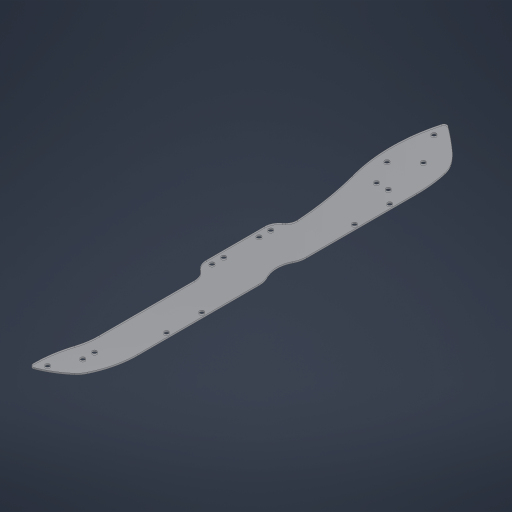
# Autodesk Inventor part: sled2
Saved by Autodesk Inventor 2024 (Build 280153000, 153)
## iProperties
Created: 2023-10-30
Part Number: sled2
Material: Polycarbonate, Smoke
Document SubType Name: Modeling
Designer: macbook
Density: 1.2 g/cm^3
Appearance: Polycarbonate - Clear(1)
Author: macbook
Autodesk Inventor part; units mm, degrees
ref_plane "YZ Plane" through (0, 0, 0) normal (1, 0, 0) x (0, 1, 0)
ref_plane "XZ Plane" through (0, 0, 0) normal (0, 1, 0) x (-1, 0, 0)
ref_plane "XY Plane" through (0, 0, 0) normal (0, 0, 1) x (1, 0, 0)
sketch "Sketch2" plane through (0, 0, 0) normal (0, 1, 0) x (-1, 0, 0)
  line L0 (25.3485, -88.9331) -> (25.3485, -76.2331)
  line L1 (25.3485, -76.2331) -> (0.0063, -76.2331)
  line L2 (0.0063, -76.2331) -> (0.0055, -63.5331)
  line L3 (0.1328, -20.6833) -> (0.1265, -35.8822)
  line L4 (38.2012, -93.5899) -> (38.2012, -99.9399)
  line L5 (12.8495, -23.9499) -> (19.1995, -23.9501)
  line L6 (19.1995, -23.9501) -> (6.4995, -23.9497)
  line L7 (25.3485, -88.9331) -> (31.6373, -88.0533)
  arc A0 (30.6963, -113.4359) -> (33.2246, -115.3327) centre (248.7957, 174.6442) ccw
  line L8 (38.2825, -88.8911) -> (38.2774, -69.8411)
  line L9 (38.2774, -69.8411) -> (44.78, -69.8393)
  arc A1 (38.3114, -113.5855) -> (38.3007, -17.4758) centre (-135.3855, -65.5498) ccw
  arc A2 (33.2246, -115.3327) -> (38.3114, -113.5855) centre (35.1695, -112.7166) ccw
  arc A3 (44.8311, -65.5299) -> (38.2642, -32.0968) centre (-43.6087, -65.5397) ccw
  line L10 (6.4995, -23.9497) -> (0.1314, -23.947)
  line L11 (0.1314, -23.947) -> (0.2658, 299.9029) construction
  line L12 (0.2658, 299.9029) -> (25.6658, 299.9029) construction
  line L13 (25.6658, 269.4446) -> (25.6658, -23.6933)
  line L14 (25.6658, -23.6933) -> (39.903, -23.6933)
  line L15 (0.2658, 299.9029) -> (-12.4342, 299.9029)
  line L16 (-12.5436, -23.9601) -> (-12.5436, -35.112)
  arc A4 (-4.3142, -80.5045) -> (7.2064, -94.0414) centre (51.9465, -44.2947) ccw
  arc A5 (-12.5436, -35.112) -> (-9.0134, -68.7415) centre (149.4014, -35.112) ccw
  arc A6 (-5.9833, -77.5413) -> (-4.3142, -80.5045) centre (19.9766, -64.8707) ccw
  arc A7 (-9.0134, -68.7415) -> (-5.9833, -77.5413) centre (28.2561, -60.8297) ccw
  arc A8 (7.2064, -94.0414) -> (30.6963, -113.4359) centre (248.7971, 174.6431) ccw
  line L17 (0.2658, 299.9029) -> (0.1867, 109.403) construction
  line L18 (0.1867, 109.403) -> (-36.5163, 109.4182)
  arc A9 (-9.714, 95.5829) -> (-9.702, 123.2303) centre (-36.5163, 109.4182) ccw
  line L19 (-12.5217, 258.1981) -> (-12.5217, 134.8616)
  line L20 (-12.5436, 83.9322) -> (-12.5436, -23.9601)
  arc A10 (-12.5217, 127.6948) -> (-12.5436, 91.1127) centre (-36.5163, 109.4182) ccw construction
  arc A11 (-12.5217, 134.8616) -> (-9.702, 123.2303) centre (12.8783, 134.8616) ccw
  arc A12 (-9.714, 95.5829) -> (-12.5436, 83.9322) centre (12.8564, 83.9322) ccw
  line L21 (25.6658, 299.9029) -> (25.6658, 331.6529)
  line L22 (25.6658, 331.6529) -> (32.0158, 331.6529)
  arc A13 (35.1908, 331.6395) -> (28.8408, 331.6529) centre (32.0158, 331.6529) ccw
  line L23 (0.2658, 299.9029) -> (0.2658, 325.3029)
  line L24 (32.0158, 331.6529) -> (30.6929, 331.6529)
  arc A14 (29.2214, 292.4497) -> (35.1908, 331.6395) centre (-92.7618, 331.0796) ccw
  line L25 (31.9383, 334.827) -> (31.4142, 334.827)
  arc A15 (31.007, 334.6634) -> (4.0007, 318.3551) centre (65.1249, 247.6497) ccw
  arc A16 (-10.3215, 302.8155) -> (-14.0041, 295.5815) centre (10.1821, 287.8234) ccw
  line L26 (-12.5217, 258.1981) -> (-12.5217, 338.0406)
  arc A17 (-2.1991, 310.3119) -> (-12.5217, 265.7661) centre (88.7553, 265.7661) ccw
  arc A18 (4.0007, 318.3551) -> (-2.1991, 310.3119) centre (20.612, 299.1399) ccw
  line L27 (0.2658, 299.9029) -> (0.2605, 287.2029)
  line L28 (0.2605, 287.2029) -> (12.9605, 287.1977)
  line L29 (0.1867, 109.403) -> (0.221, 191.953)
  line L30 (0.221, 191.953) -> (-7.7165, 191.9562)
  line L31 (0.1867, 109.403) -> (0.1525, 26.853)
  line L32 (0.1525, 26.853) -> (-7.785, 26.853)
  line L33 (-7.785, 26.853) -> (-7.785, -11.247)
  line L34 (-7.7165, 191.9562) -> (-7.7165, 230.0562)
  arc A19 (25.6658, 282.6329) -> (27.2405, 286.6766) centre (-92.7618, 331.0796) ccw
  arc A20 (29.2214, 292.4497) -> (25.6658, 269.4446) centre (101.8658, 269.4446) ccw
  line L35 (25.6658, 109.403) -> (32.0158, 109.403)
  line L36 (32.0158, 109.403) -> (32.0158, 90.353)
  line L37 (32.0158, 90.353) -> (32.0158, 77.653)
  line L38 (32.0158, 109.403) -> (32.0158, 128.453)
  line L39 (32.0158, 128.453) -> (32.0158, 141.153)
  line L40 (32.0158, 109.403) -> (38.3658, 109.403)
  line L41 (38.3658, 109.403) -> (38.3658, 141.153)
  arc A21 (38.3658, 141.153) -> (32.0778, 153.6114) centre (22.8798, 141.153) ccw
  arc A22 (25.6658, 83.9658) -> (25.6658, 78.268) centre (416.3302, 81.1169) ccw
  arc A23 (26.6118, 53.7976) -> (38.3007, -17.4758) centre (416.3302, 81.1169) ccw
  arc A24 (25.6658, 166.3155) -> (32.0778, 153.6114) centre (41.457, 166.3155) ccw
  line L42 (38.3658, 109.403) -> (38.3658, 77.653)
  arc A25 (32.0778, 65.1945) -> (38.3658, 77.653) centre (22.8798, 77.653) ccw
  arc A26 (32.0778, 65.1945) -> (30.3394, 63.7048) centre (41.457, 52.4904) ccw
  arc A27 (30.3394, 63.7048) -> (26.6118, 53.7976) centre (39.2807, 54.6857) ccw
  line L43 (25.6658, 299.9029) -> (25.6658, 325.3029)
  line L44 (12.9605, 287.1977) -> (12.9605, 299.8977)
  point P0 (0.0775, -39.6857)
  point P1 (12.8012, -68.1967)
  point P2 (37.0807, -118.1599)
  point P3 (33.0954, -49.1463)
  point P4 (33.0954, -99.9463)
  point P5 (33.0954, -99.9463)
  point P6 (33.0954, -49.1463)
  point P7 (30.6993, 334.5421)
  point P8 (25.6658, 160.9899)
  point P9 (25.6658, 57.8161)
  point P10 (25.6658, 52.4904)
  point P11 (26.3876, 57.21)
  dimension "d3" = 12.7
  dimension "d5" = 12.7
  dimension "d37" = 6.35
  dimension "d54" = 6.35
  dimension "d55" = 25.4
  dimension "d58" = 19.05
  dimension "d82" = 323.85
  dimension "d83" = 25.4
  dimension "d84" = 12.7
  dimension "d85" = 38.1
  dimension "d86" = 190.5
  dimension "d87" = 60.325
  dimension "d88" = 36.703
  dimension "d89" = 25.4
  dimension "d93" = 6.35
  dimension "d94" = 6.35
  dimension "d95" = 31.75
  dimension "d97" = 25.4
  dimension "d99" = 25.4
  dimension "d102" = 25.4
  dimension "d103" = 12.7
  dimension "d104" = 12.7
  dimension "d105" = 82.55
  dimension "d106" = 7.9375
  dimension "d107" = 82.55
  dimension "d108" = 38.1
  dimension "d109" = 38.1
  dimension "d110" = 76.2
  dimension "d111" = 6.35
  dimension "d112" = 19.05
  dimension "d113" = 12.7
  dimension "d114" = 19.05
  dimension "d115" = 12.7
  dimension "d116" = 6.35
  dimension "d117" = 31.75
  dimension "d118" = 12.7
  dimension "d119" = 12.7
  constraints: 90 end point, 67 point on circle, 28 centre point, 22 tangent, 21 point on line, 18 coincident, 13 perpendicular, 10 vertical, 6 horizontal, 5 symmetric about line, 1 equal radius, 1 midpoint, 2 other
  measures "d3" distance of L0.start L0.end
  measures "d5" distance of L1.end L2.end
  measures "d37" distance of L5.start L5.end
  measures "d54" distance of L0.start L7.end
  measures "d55" distance of L7.end A0.start
  measures "d58" distance of L8.start L8.end
  measures "d82" distance of L10.end L11.end
  measures "d83" distance of L11.end L12.end
  measures "d84" distance of L11.end L15.end
  measures "d85" radius of A7
  measures "d86" distance of L11.end L17.end
  measures "d87" diameter of A9
  measures "d88" distance of L17.end L18.end
  measures "d89" radius of A11
  measures "d93" distance of L21.end L22.end
  measures "d94" diameter of A13
  measures "d95" distance of L12.end L21.end
  measures "d97" distance of L11.end L23.end
  measures "d99" radius of A16
  measures "d102" radius of A18
  measures "d103" distance of L11.end L27.end
  measures "d104" distance of L27.end L28.end
  measures "d105" distance of L17.end L29.end
  measures "d106" distance of L29.end L30.end
  measures "d107" distance of L17.end L31.end
  measures "d108" distance of L33.start L33.end
  measures "d109" distance of L34.start L34.end
  measures "d110" radius of A20
  measures "d111" distance of L35.start L35.end
  measures "d112" distance of L35.end L36.end
  measures "d113" distance of L36.end L37.end
  measures "d114" distance of L35.end L38.end
  measures "d115" distance of L38.end L39.end
  measures "d116" distance of L40.start L40.end
  measures "d117" distance of L40.end L41.end
  measures "d118" radius of A27
  measures "d119" distance of L44.start L44.end
extrude "Extrusion1" add sketch "Sketch2" along normal blind 1.5875 contours A8 A4 A6 A7 A5 L16 L20 A12 A9 A11 L19 L26 A17 L15 L23 A18 A15 A13 A14 A20 L13 A22 L14 A1 A2 A0 | L14 L13 L35 L40 L42 A25 A26 A27 A23 A1 | A22 L13 | L13 A24 A21 L41 L40 L35 | A17 A18 L23 L15 | A15 A13
hole "Hole3" at (-6.4995, 0, -23.9497) at (-19.1995, 0, -23.9501) at (-12.8012, 0, -68.1967) at (-33.0954, 0, -49.1463) at (-33.0954, 0, -99.9463) at (-12.9605, 0, 287.1977) at (7.7165, 0, 191.9562) at (7.785, 0, 26.853) at (7.785, 0, -11.247) at (7.7165, 0, 230.0562) at (-32.0158, 0, 141.153) at (-32.0158, 0, 128.453) at (-32.0158, 0, 90.353) at (-32.0158, 0, 77.653) at (-25.6658, 0, 325.3029) at (-12.9605, 0, 299.8977) direction (0, 1, 0) diameter 4.7625 end through all
body "Solid1"
